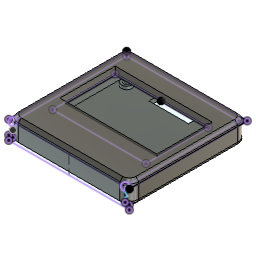
OLED+Display+Case (Autodesk Fusion 360 design; units mm, degrees)
Autodesk Fusion 360 part; units mm, degrees
sketch "Screen PCB" plane through (0, 0, 0) normal (0, 0, 1) x (1, 0, 0)
  line L0 (0, 0) -> (27.4, 0)
  line L1 (27.4, 0) -> (27.4, 27.8)
  line L2 (27.4, 27.8) -> (0, 27.8)
  line L3 (0, 27.8) -> (0, 0)
  line L4 (8.7, 27.8) -> (18.7, 27.8)
  line L5 (18.7, 27.8) -> (18.7, 25.4)
  line L6 (18.7, 25.4) -> (8.7, 25.4)
  line L7 (8.7, 25.4) -> (8.7, 27.8)
  line L8 (1.4, 23.3) -> (26, 23.3)
  line L9 (26, 23.3) -> (26, 6.9)
  line L10 (26, 6.9) -> (1.4, 6.9)
  line L11 (1.4, 6.9) -> (1.4, 23.3)
  line L12 (13.7, 6.9) -> (13.7, 0) construction
  circle A0 centre (2, 2) radius 1
  circle A1 centre (25.4, 2) radius 1
  circle A2 centre (2, 25.8) radius 1
  circle A3 centre (25.4, 25.8) radius 1
  point P0 (13.7, 6.9)
  point P1 (13.7, 0)
  dimension "d1" = 27.4
  dimension "d2" = 27.8
  dimension "d14" = 10
  dimension "d15" = 2.4
  dimension "d16" = 24.6
  dimension "d17" = 16.4
  dimension "d18" = 4.5
  dimension "d19" = 1.4
  dimension "d20" = 6.9
  dimension "d21" = 2
  dimension "d22" = 2
  dimension "d23" = 2
  dimension "d26" = 23.4
  dimension "d27" = 23.8
  constraint horizontal L0
  constraint vertical L1
  constraint horizontal L2
  constraint vertical L3
  constraint coincident L0.start L3.end
  constraint horizontal L4
  constraint vertical L5
  constraint horizontal L6
  constraint vertical L7
  constraint midpoint L2 L4
  constraint horizontal L8
  constraint vertical L9
  constraint horizontal L10
  constraint vertical L11
  constraint midpoint L10 P0
  constraint midpoint L0 P1
  constraint coincident P0 L12.start
  constraint coincident P1 L12.end
  constraint perpendicular L10 L12
  measures "d1" distance of L0.start L0.end
  measures "d2" distance of L0.start L2.end
  measures "d14" distance of L4.start L4.end
  measures "d15" distance of L4.start L6.end
  measures "d16" distance of L8.start L8.end
  measures "d17" distance of L8.start L10.end
  measures "d18" distance of L2 L8
  measures "d19" distance of L3 L10.end
  measures "d20" distance of L0 L9.end
  measures "d21" diameter of A0
  measures "d22" distance of L0 A0.centre
  measures "d23" distance of L3 A0.centre
sketch "Case Base" plane through (0, 0, 0) normal (0, 0, 1) x (1, 0, 0)
  line L0 (27.4, 27.8) -> (0, 27.8)
  line L1 (27.4, 0) -> (27.4, 27.8)
  line L2 (0, 27.8) -> (0, 0)
  line L3 (0, 0) -> (27.4, 0)
  line L4 (-0.2, -0.2) -> (27.6, -0.2)
  line L5 (27.6, -0.2) -> (27.6, 28)
  line L6 (27.6, 28) -> (-0.2, 28)
  line L7 (-0.2, 28) -> (-0.2, -0.2)
  circle A0 centre (2, 25.8) radius 1
  circle A1 centre (25.4, 25.8) radius 1
  circle A2 centre (25.4, 2) radius 1
  circle A3 centre (2, 2) radius 1
  circle A4 centre (2, 25.8) radius 0.8
  circle A5 centre (25.4, 25.8) radius 0.8
  circle A6 centre (25.4, 2) radius 0.8
  circle A7 centre (2, 2) radius 0.8
  line L8 (28.5, 28.9) -> (-1.1, 28.9)
  line L9 (-1.1, 28.9) -> (-1.1, -1.1)
  line L10 (-1.1, -1.1) -> (28.5, -1.1)
  line L11 (28.5, -1.1) -> (28.5, 28.9)
  circle A8 centre (2, 25.8) radius 1.4
  circle A9 centre (25.4, 25.8) radius 1.4
  circle A10 centre (25.4, 2) radius 1.4
  circle A11 centre (2, 2) radius 1.4
  line L12 (18.7, 27.8) -> (18.7, 25.4)
  line L13 (18.7, 25.4) -> (8.7, 25.4)
  line L14 (8.7, 25.4) -> (8.7, 27.8)
  line L15 (8.7, 27.8) -> (18.7, 27.8)
  line L16 (8.5, 28) -> (18.9, 28)
  line L17 (18.9, 28) -> (18.9, 25.2)
  line L18 (18.9, 25.2) -> (8.5, 25.2)
  line L19 (8.5, 25.2) -> (8.5, 28)
  line L20 (-2.2, 30) -> (29.6, 30)
  line L21 (29.6, 30) -> (29.6, -1.1)
  line L22 (29.6, -1.1) -> (-2.2, -1.1)
  line L23 (-2.2, -1.1) -> (-2.2, 30)
  point P0 (2, 25.8)
  dimension "d28" = 0.2
  dimension "d33" = 1.1
  dimension "d37" = 0.4
  dimension "d38" = 0.4
  dimension "d39" = 0.4
  dimension "d40" = 0.4
  dimension "d53" = 1.1
  dimension "d54" = 1.1
  constraint horizontal L20
  constraint vertical L21
  constraint horizontal L22
  constraint vertical L23
  constraint midpoint L10 L22
  measures "d53" distance of L8.end L23
  measures "d54" vertical distance of L8.end L20.start
extrude "Extrude3" add sketch "Case Base" against normal blind 1.2 contours L0 L1 L2 L3 L4 L5 L6 L7 L17 L19 | L0 L1 L2 L3 L17 L18 L19 | A0 | A1 | A2 | A3 | A4 | A5 | A6 | A7 | L8 L9 L10 L11 L22 | L8 L9 L11 L20 L21 L22 L23 | A8 | A9 | A10 | A11 makes body 1
extrude "Extrude1" add sketch "Case Base" along normal blind 0.8 contours A0 | A1 | A2 | A3 | A8 | A9 | A10 | A11 bodies 1
extrude "Extrude2" add sketch "Case Base" along normal blind 2 contours A4 | A5 | A6 | A7 bodies 1
extrude "Extrude4" add sketch "Case Base" along normal blind 3.6 contours L8 L9 L10 L11 L22 bodies 1
fillet "Fillet1" radius 0.5 4 faces at (1.8444, 25.6186, 2) (25.5333, 26.1881, 2) (2.4109, 1.7341, 2) (25.6548, 1.9214, 2) on bodies 1
copy_body "Body->Comp1" bodies 1 removing the originals makes body 2 in component "Base"
sketch "Sketch3" plane through (0, -1.1, 0) normal (0, -1, 0) x (1, 0, 0)
  line L0 (28.5, 3.6) -> (-1.1, 3.6)
  line L1 (29.6, 0) -> (28.5, 0)
  line L2 (28.5, 0) -> (28.5, 3.6)
  line L3 (-1.1, 3.6) -> (-1.1, 0)
  line L4 (-1.1, 0) -> (-2.2, 0)
  line L5 (-2.2, 0) -> (-2.2, -1.2)
  line L6 (-2.2, -1.2) -> (29.6, -1.2)
  line L7 (29.6, -1.2) -> (29.6, 0)
  line L8 (-1.1, 1.7) -> (-1.7, 1.7) construction
  line L9 (-1.1, 1.7) -> (-1.1, 2.3)
  line L10 (-1.1, 2.3) -> (-1.7, 1.7)
  line L11 (-1.1, 1.7) -> (-1.1, 1.1)
  line L12 (-1.1, 1.1) -> (-1.7, 1.7)
  line L13 (13.7, 3.6) -> (13.7, -1.2) construction
  line L14 (28.5, 1.7) -> (28.5, 2.3)
  line L15 (28.5, 1.7) -> (28.5, 1.1)
  line L16 (28.5, 2.3) -> (29.1, 1.7)
  line L17 (28.5, 1.7) -> (29.1, 1.7) construction
  line L18 (28.5, 1.1) -> (29.1, 1.7)
  dimension "d58" = 0.6
  dimension "d59" = 0.6
  dimension "d60" = 0.6
  constraint coincident L3 L8.start
  constraint perpendicular L3 L8
  constraint perpendicular L8 L9
  constraint perpendicular L8 L11
  constraint midpoint L0 L13.start
  constraint midpoint L6 L13.end
  constraint symmetric L8.start L13 L14.start
  constraint symmetric L8.end L13 L16.end
  constraint symmetric L9.end L13 L14.end
  constraint symmetric L11.end L13 L15.end
  measures "d58" distance of L8.start L8.end
  measures "d59" distance of L8.start L9.end
  measures "d60" distance of L8.start L11.end
fillet "Fillet1'" radius 2.5 4 edges at (-2.2, -1.1, -0.6) (29.6, -1.1, -0.6) (29.6, 30, -0.6) (-2.2, 30, -0.6) on bodies 2 in component "Base"
chamfer "Chamfer1" distance 0.8 angle 45 8 edges at (13.7, -1.1, -1.2) (-1.4678, -0.3678, -1.2) (-2.2, 14.45, -1.2) (-1.4678, 29.2678, -1.2) (13.7, 30, -1.2) (28.8678, 29.2678, -1.2) (29.6, 14.45, -1.2) (28.8678, -0.3678, -1.2) on bodies 2 in component "Base"
extrude "Extrude1'" add sketch "Sketch3" along normal blind -25.8 and the other way blind 4 contours L2 L14 L15 L16 L18 | L3 L9 L10 L11 L12 bodies 2 in component "Base"
sketch "Sketch1" plane through (0, 0, 3.6) normal (0, 0, 1) x (-1, 0, 0) in component "Lid"
  line L0 (0.2, 0.2) -> (0.2, -28)
  line L1 (0.2, -28) -> (-27.6, -28)
  line L2 (-27.6, -28) -> (-27.6, 0.2)
  line L3 (-27.6, 0.2) -> (0.2, 0.2)
  arc A0 (-27.1, 1.1) -> (-28.5, 0.6712) centre (-27.1, -1.4) ccw
  line L4 (-28.5, 0.6712) -> (-28.5, -28.9)
  line L5 (-28.5, -28.9) -> (1.1, -28.9)
  line L6 (1.1, -28.9) -> (1.1, 0.6712)
  arc A1 (1.1, 0.6712) -> (-0.3, 1.1) centre (-0.3, -1.4) ccw
  line L7 (-0.3, 1.1) -> (-27.1, 1.1)
  line L8 (-29.6, 1.1) -> (2.2, 1.1)
  line L9 (2.2, 1.1) -> (2.2, -30)
  line L10 (2.2, -30) -> (-29.6, -30)
  line L11 (-29.6, -30) -> (-29.6, 1.1)
  line L12 (1.1, -28.9) -> (1.1, 1.1)
  line L13 (-28.5, -28.9) -> (1.1, -28.9)
  line L14 (-28.5, 1.1) -> (-28.5, -28.9)
  line L15 (2.2, -30) -> (-29.6, -30)
  line L16 (-29.6, -30) -> (-29.6, 1.1)
  line L17 (-29.6, 1.1) -> (2.2, 1.1)
  line L18 (2.2, 1.1) -> (2.2, -30)
  line L19 (-26, -6.9) -> (-1.4, -6.9)
  line L20 (-1.4, -6.9) -> (-1.4, -23.3)
  line L21 (-1.4, -23.3) -> (-26, -23.3)
  line L22 (-26, -23.3) -> (-26, -6.9)
  line L23 (-1.7, -23.1) -> (-25.7, -23.1)
  line L24 (-25.7, -23.1) -> (-25.7, -10.1)
  line L25 (-25.7, -10.1) -> (-1.7, -10.1)
  line L26 (-1.7, -10.1) -> (-1.7, -23.1)
  line L27 (-13.7, -23.3) -> (-13.7, -23.1) construction
  point P0 (-13.7, -23.1)
  point P1 (-13.7, -23.3)
  dimension "d65" = 24
  dimension "d66" = 13
  dimension "d67" = 0.2
  constraint horizontal L15
  constraint vertical L16
  constraint horizontal L17
  constraint vertical L18
  constraint coincident L8.start L11.end
  constraint coincident L9.end L10.start
  constraint horizontal L23
  constraint vertical L24
  constraint horizontal L25
  constraint vertical L26
  constraint midpoint L23 P0
  constraint midpoint L21 P1
  constraint coincident P1 L27.start
  constraint coincident P0 L27.end
  constraint vertical L27
  measures "d65" distance of L23.start L23.end
  measures "d66" distance of L23.start L25.end
  measures "d67" distance of P1 P0
extrude "Extrude1''" add sketch "Sketch1" against normal blind 3.6 separate body contours L4 L5 L6 L8 L9 L10 L11 L12 L13 L14 L15 L16 L17 L18 makes body 3 in component "Lid"
extrude "Extrude2'" add sketch "Sketch1" along normal blind 1.2 contours L0 L1 L2 L3 | A0 L4 L5 L6 A1 L7 L8 L12 L13 L14 L17 | A0 L8 L14 L17 | L4 L5 L6 L8 L9 L10 L11 L12 L13 L14 L15 L16 L17 L18 | A1 L8 L12 L17 | L19 L20 L21 L22 bodies 3 in component "Lid"
extrude "Extrude3'" cut sketch "Sketch3" along normal blind -25.8 and the other way blind 4 contours L2 L14 L15 L16 L18 | L3 L9 L10 L11 L12 bodies 3 in component "Lid"
fillet "Fillet1''" radius 2.5 4 edges at (29.6, -1.1, 2.4) (-2.2, -1.1, 2.4) (29.6, 30, 2.4) (-2.2, 30, 2.4) on bodies 3 in component "Lid"
chamfer "Chamfer1'" distance 0.8 angle 45 1 faces at (17.7, 2.6333, 4.8) on bodies 3 in component "Lid"
move_face "OffsetFaces1" offset -0.1 4 faces at (-1.3, 10.1667, 2.1) (-1.3, 10.1667, 1.3) (-1.3, 2.9, 1.7) (-1.3, 24.7, 1.7) on bodies 3 in component "Lid"
move_face "OffsetFaces2" offset -0.1 4 faces at (28.7, 24.7, 1.7) (28.7, 10.1667, 1.3) (28.7, 10.1667, 2.1) (28.7, 2.9, 1.7) on bodies 3 in component "Lid"
component "Base" placed x (1, 0, 0) y (0, 1, 0) z (0, 0, 1) at (0, 0, 0)
component "Lid" placed x (1, 0, 0) y (0, 1, 0) z (0, 0, 1) at (0, 0, 0)
equation "d1 = board_width"
equation "d2 = board_height"
equation "board_width = 27.4 mm"
equation "board_height = 27.8 mm"
equation "tollerance = 0.2 mm"
equation "board_depth = 1.2 mm"
equation "hole_diameter = 2.0 mm"
equation "hole_to_edge = 1.0 mm"
equation "screen_width = 24.6 mm"
equation "screen_height = 16.4 mm"
equation "screen_and_board_depth = 2.8 mm"
equation "pins_width = 10.0 mm"
equation "pins_height = 2.4 mm"
equation "d14 = pins_width"
equation "d15 = pins_height"
equation "d16 = screen_width"
equation "d17 = screen_height"
equation "d21 = hole_diameter"
equation "d22 = hole_to_edge + ( hole_diameter / 2 )"
equation "d23 = hole_to_edge + ( hole_diameter / 2 )"
equation "d26 = board_width - hole_diameter - ( 2 * hole_to_edge )"
equation "d27 = board_height - hole_diameter - ( 2 * hole_to_edge )"
equation "d28 = tollerance"
equation "d29 = -tollerance"
equation "d30 = -tollerance"
equation "d31 = -tollerance"
equation "d32 = -tollerance"
equation "d33 = inner_wall_width + tollerance"
equation "inner_wall_width = 0.9 mm"
equation "outer_wall_width = 1.1 mm"
equation "base_thickness = 1.2 mm"
equation "d41 = -tollerance"
equation "riser = 0.8 mm"
equation "d43 = riser"
equation "d45 = riser + board_depth"
equation "d47 = -base_thickness"
equation "d49 = riser + screen_and_board_depth"
equation "d52 = hole_diameter / 4"
equation "d53 = outer_wall_width"
equation "d54 = outer_wall_width"
equation "d61 = -( board_height - inner_wall_width - outer_wall_width )"
equation "d63 = ( inner_wall_width + outer_wall_width ) * 2"
equation "d68 = -( screen_and_board_depth + riser )"
equation "d70 = board_depth"
equation "d72 = -( board_height - inner_wall_width - outer_wall_width )"
equation "d74 = ( inner_wall_width + outer_wall_width ) * 2"
equation "d79 = -tollerance / 2"
equation "d80 = -tollerance / 2"
